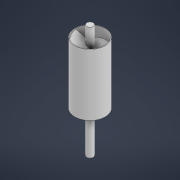
# Autodesk Inventor part: 螺旋
Saved by Autodesk Inventor 2021 (Build 250183000, 183)
## iProperties
Created: 2020-12-30
Part Number: 螺旋
Material: 一般
Document SubType Name: Modeling
Designer: zihon
Density: 1 g/cm^3
Appearance: 預設
Author: zihon
Autodesk Inventor part; units mm, degrees
ref_plane "YZ Plane" through (0, 0, 0) normal (1, 0, 0) x (0, 1, 0)
ref_plane "XY Plane" through (0, 0, 0) normal (0, 0, 1) x (1, 0, 0)
sketch "草圖1" plane through (0, 0, 0) normal (0, 0, 1) x (1, 0, 0)
  line L0 (-42.6, 145.5648) -> (-45.1015, 136.229)
  line L1 (-45.1015, 136.229) -> (-11.2941, 127.1704)
  line L2 (-11.2941, 127.1704) -> (-10, 132)
  line L3 (-10, 132) -> (-43.8074, 141.0587)
  line L4 (-65.9414, 0) -> (65.9414, 0) projected
  line L5 (0, 123.0754) -> (0, 149.313) projected
  line L6 (-10, 132) -> (-10, 126.8236)
  line L7 (-10, 126.8236) -> (-11.2941, 127.1704)
  line L8 (-43.8074, 141.0587) -> (-43.8074, 135.8823)
  dimension "d2" = 35
  dimension "d4" = 5
  dimension "d5" = 10
  dimension "d7" = 15
  dimension "d19" = 45.1015
  dimension "d24" = 132
  dimension "d25" = 126.8236
  constraints: 14 end point, 4 perpendicular, 2 point on line, 2 vertical
  measures "d2" distance of L2.end L3.end
  measures "d4" distance of L1.end L2.end
  measures "d5" distance from line of L5 L2.end
  measures "d7" angle of L4 L1
  measures "d19" distance from line of L5 L0.end
  measures "d24" distance from line of L4 L2.end
  measures "d25" distance from line of L4 L6.end
coil "螺旋1" sketch "草圖1" operation add axis through (0, -10, 0) along (0, 1, 0) pitch 35 turns 5 hand left contours L3 L2 L1 L8 | L6 L7 L2
sketch "草圖2" plane through (0, 0, 0) normal (0, 1, 0) x (-1, 0, 0)
  line L0 (43.8074, 0) -> (10, 0) projected
  circle A0 centre (0, 0) radius 10
  constraints: 1 coincident, 1 horizontal alignment, 2 other
extrude "擠出1" add sketch "草圖2" along normal blind 350
ref_plane "工作平面1" through (0, 126.824, 0) normal (0, 1, 0) x (-1, 0, 0)
sketch "草圖3" plane through (0, 126.824, 0) normal (0, 1, 0) x (-1, 0, 0)
  circle A0 centre (0, 0) radius 45.101
  circle A1 centre (0, 0) radius 47.101
  dimension "d20" = 90.202
  dimension "d21" = 2
  constraints: 2 centre point, 1 coincident
  measures "d20" diameter of A0
  measures "d21" radial gap between concentric circles of A0 A1
extrude "擠出3" add sketch "草圖3" along normal blind 190
